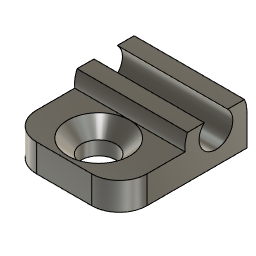
Reed Switch Holder v2 (Autodesk Fusion 360 design; units mm, degrees)
Autodesk Fusion 360 part; units mm, degrees
sketch "Sketch1" plane through (0, 0, 0) normal (1, 0, 0) x (0, 1, 0)
  circle A0 centre (0, 0) radius 1.225
  circle A1 centre (0, 0) radius 2.25
  line L0 (0, -2.25) -> (-7, -2.25)
  line L1 (-7, -2.25) -> (-7, -0.25)
  line L2 (-7, -0.25) -> (0, -0.25)
  line L3 (0, -0.25) -> (0, -2.25)
  line L4 (-4.9672, 4.6123) -> (6.1553, 4.6123)
  line L5 (6.1553, 4.6123) -> (6.1553, 0.8852)
  line L6 (6.1553, 0.8852) -> (-4.9672, 0.8852)
  line L7 (-4.9672, 0.8852) -> (-4.9672, 4.6123)
  line L8 (0, -2.25) -> (2.25, -2.25)
  line L9 (2.25, -2.25) -> (2.25, 0)
  line L10 (2.25, 0) -> (0, 0)
  line L11 (0, 0) -> (0, -2.25)
  dimension "d1" = 2.45
  dimension "d2" = 4.5
  dimension "d3" = 7
  dimension "d4" = 2
  dimension "d5" = 2.25
  dimension "d6" = 2.25
  constraint coincident A0.centre A1.centre
  constraint horizontal L0
  constraint vertical L1
  constraint horizontal L2
  constraint vertical L3
  constraint coincident A1 L0.start
  constraint horizontal L4
  constraint vertical L5
  constraint horizontal L6
  constraint vertical L7
  constraint horizontal L8
  constraint vertical L9
  constraint horizontal L10
  constraint vertical L11
  measures "d1" diameter of A0
  measures "d2" diameter of A1
  measures "d3" distance of L0.start L0.end
  measures "d4" distance of L0.start L2.end
  measures "d5" distance of L0.start L8.end
  measures "d6" distance of L0.start A0.centre
extrude "Extrude1" add sketch "Sketch1" along normal blind 8 contours A0 A1 L3 L10 L11 | A0 A1 L6 L10 | A0 A1 L2 L3 L11 | A1 L8 L9 | A0 A1 L2 L6 | A1 L0 L1 L2
sketch "Sketch2" plane through (0, 0, 0) normal (0, 0, 1) x (1, 0, 0)
  circle A0 centre (4, -4.5) radius 1.25
  dimension "d9" = 2.5
  measures "d9" diameter of A0
extrude "Extrude2" cut sketch "Sketch2" against normal blind 6.5
chamfer "Chamfer1" distance 1 angle 45 1 edges at (2.8346, -4.048, -0.25)
fillet "Fillet1" radius 2 2 edges at (0, -7, -1.25) (8, -7, -1.25)
